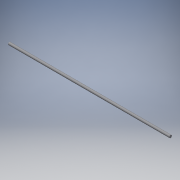
# Autodesk Inventor part: Bore
Saved by Autodesk Inventor 2019.4 (Build 234330000, 330)
## iProperties
Created: 2020-01-10
Part Number: Bore
Material: Generic
Document SubType Name: Modeling
Designer: Mark
Mass: 83.0134 g
Surface Area: 278.973 cm^2
Volume: 83.0134 cm^3
Density: 1 g/cm^3
Appearance: Default
Author: Mark
Autodesk Inventor part; units mm, degrees
ref_plane "YZ Plane" through (0, 0, 0) normal (1, 0, 0) x (0, 1, 0)
ref_plane "XZ Plane" through (0, 0, 0) normal (0, 1, 0) x (-1, 0, 0)
ref_plane "XY Plane" through (0, 0, 0) normal (0, 0, 1) x (1, 0, 0)
sketch "Sketch1" plane through (0, 0, 0) normal (1, 0, 0) x (0, 1, 0)
  circle A0 centre (0, 0) radius 6
  dimension "d0" = 12
  constraints: 1 centre point, 1 coincident
  measures "d0" diameter of A0
extrude "Extrusion1" add sketch "Sketch1" along normal blind 734
body "Solid1"
